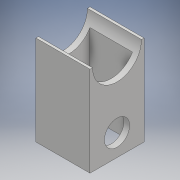
# Autodesk Inventor part: 左右に飛び出すパイプ
Saved by Autodesk Inventor 2018 (Build 220112000, 112)
## iProperties
Created: 2017-09-10
Part Number: 左右に飛び出すパイプ
Material: 一般
Document SubType Name: Modeling
Designer: Kenta
Density: 1 g/cm^3
Appearance: 既定
Author: Kenta
Autodesk Inventor part; units mm, degrees
ref_plane "YZ Plane" through (0, 0, 0) normal (1, 0, 0) x (0, 1, 0)
ref_plane "XZ Plane" through (0, 0, 0) normal (0, 1, 0) x (-1, 0, 0)
ref_plane "XY Plane" through (0, 0, 0) normal (0, 0, 1) x (1, 0, 0)
sketch "スケッチ5" plane through (0, 0, 0) normal (0, 0, 1) x (1, 0, 0)
  line L0 (-15, 15) -> (15, 15)
  line L1 (15, 15) -> (15, -15)
  line L2 (15, -15) -> (-15, -15)
  line L3 (-15, -15) -> (-15, 15)
  line L4 (-15, 15) -> (15, -15) construction
  line L5 (15, 15) -> (-15, -15) construction
  line L6 (11.8, 11.8) -> (-11.8, 11.8)
  line L7 (-11.8, 11.8) -> (-11.8, -11.8)
  line L8 (-11.8, -11.8) -> (11.8, -11.8)
  line L9 (11.8, -11.8) -> (11.8, 11.8)
  point P0 (0, 0)
  dimension "d15" = 30
  dimension "d16" = 30
  dimension "d17" = 3.2
  constraints: 20 end point, 4 parallel, 2 midpoint, 2 perpendicular, 1 horizontal, 3 other
  measures "d15" distance of L1.end L2.end
  measures "d16" distance of L0.end L1.end
  measures "d17" distance between parallel lines of L0 L6
extrude "押し出し3" add sketch "スケッチ5" against normal blind 50
sketch "スケッチ6" plane through (0, 0, 0) normal (1, 0, 0) x (0, 1, 0)
  circle A0 centre (0, 0) radius 13.6
  dimension "d20" = 27.2
  constraints: 1 centre point, 1 coincident
  measures "d20" diameter of A0
extrude "押し出し4" cut sketch "スケッチ6" along normal mid plane 30
sketch "スケッチ7" plane through (0, 0, 0) normal (1, 0, 0) x (0, 1, 0)
  line L0 (15, -50) -> (-15, -50) projected
  circle A0 centre (0, -38) radius 7
  point P0 (0, 0)
  dimension "d23" = 12
  dimension "d24" = 14
  constraints: 1 centre point, 1 coincident
  measures "d23" distance from line of L0 point (0, -38)
  measures "d24" diameter of A0
extrude "押し出し5" cut sketch "スケッチ7" along normal mid plane 30
